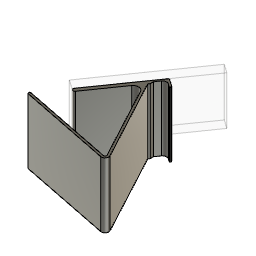
Mobilstativ v1 (Autodesk Fusion 360 design; units mm, degrees)
Autodesk Fusion 360 part; units mm, degrees
sketch "Sketch1" plane through (0, 0, 0) normal (0, 0, 1) x (1, 0, 0) in component "phone"
sketch "Sketch2" plane through (0, 0, 0) normal (0, 0, 1) x (1, 0, 0) in component "phone"
  line L0 (0, 0) -> (-28.507, 0)
  line L1 (-28.507, 0) -> (-28.507, 300.0044)
  line L2 (-28.507, 300.0044) -> (0, 300.0044)
  line L3 (0, 300.0044) -> (0, 0)
  line L4 (0, 50) -> (0, 0)
  constraint horizontal L0
  constraint vertical L1
  constraint horizontal L2
  constraint coincident L0.start L3.end
extrude "Extrude1" add sketch "Sketch2" along normal blind 40 makes body 1 in component "phone"
extrude "Extrude2" add 1 faces at (-19.0047, 116.6681, 40) along direction (0, 0, 1) blind 90 on bodies 1 bodies 1 in component "phone"
sketch "Sketch1 (2)" plane through (9.6747, 10.4809, 148.0794) normal (0, 0, 1) x (-1, 0, 0) in component "stativ"
  line L0 (68.4004, 125.7769) -> (-103.6751, -119.9723)
  line L1 (-103.6751, -119.9723) -> (-80.3235, -136.3232)
  line L2 (-80.3235, -136.3232) -> (91.7519, 109.4259)
  line L3 (91.7519, 109.4259) -> (68.4004, 125.7769)
  line L4 (65.5325, 121.6811) -> (-17.6373, 2.9023)
  line L5 (-22.9286, 12.7801) -> (-139.9865, 231.3065)
  line L6 (-129.2068, 245.8335) -> (115.8461, 196.73)
  line L7 (-17.6373, 2.9023) -> (-38.6827, -27.1535)
  line L8 (-41.4681, -27.6447) -> (-61.6426, -13.5184)
  line L9 (-25.8289, -0.0792) -> (-34.7484, -12.8175)
  line L10 (-50.0684, -15.5189) -> (-57.9556, -9.9962)
  arc A0 (-129.2068, 245.8335) -> (-139.9865, 231.3065) centre (-131.1715, 236.0284) ccw
  line L11 (-30.5905, 39.7902) -> (-134.6975, 234.1396)
  arc A1 (-130.3856, 239.9504) -> (-134.6975, 234.1396) centre (-131.1715, 236.0284) ccw
  line L12 (-130.3856, 239.9504) -> (114.6673, 190.847)
  line L13 (64.3046, 128.6448) -> (64.3046, 128.6448)
  line L14 (117.0212, 192.415) -> (117.4142, 194.376)
  arc A2 (114.6673, 190.847) -> (117.0212, 192.415) centre (115.0602, 192.808) ccw
  arc A3 (117.4142, 194.376) -> (115.8461, 196.73) centre (115.4532, 194.769) ccw
  arc A4 (64.3046, 128.6448) -> (57.341, 127.4169) centre (61.4367, 124.549) ccw
  arc A5 (65.5325, 121.6811) -> (64.3046, 128.6448) centre (61.4367, 124.549) ccw
  line L15 (-25.8289, 8.6381) -> (-25.8289, -0.0792)
  line L16 (-61.8882, -12.1256) -> (-60.7411, -10.4873)
  line L17 (57.341, 127.4169) -> (-5.0807, 38.2694)
  line L18 (-22.9286, 12.7801) -> (-25.8289, 8.6381)
  arc A6 (-50.0684, -15.5189) -> (-34.7484, -12.8175) centre (-43.759, -6.5082) ccw
  arc A7 (-41.4681, -27.6447) -> (-38.6827, -27.1535) centre (-40.321, -26.0064) ccw
  arc A8 (-57.9556, -9.9962) -> (-60.7411, -10.4873) centre (-59.1027, -11.6345) ccw
  arc A9 (-61.8882, -12.1256) -> (-61.6426, -13.5184) centre (-61.0691, -12.6992) ccw
  arc A10 (-30.5905, 39.7902) -> (-5.0807, 38.2694) centre (-17.368, 46.8731) ccw
  dimension "d9" = 10
  dimension "d10" = 2
  dimension "d11" = 5
  dimension "d12" = 11
  dimension "d13" = 2
  dimension "d14" = 2
  dimension "d15" = 1
  dimension "d16" = 15
  constraint midpoint L0 L4.end
  constraint perpendicular L7 L8
  constraint tangent L5 A0
  constraint tangent L6 A0
  constraint perpendicular L6 L14
  constraint concentric A0 A1
  constraint tangent L11 A1
  constraint tangent A1 L12
  constraint tangent L12 A2
  constraint tangent L14 A2
  constraint tangent L6 A3
  constraint tangent L14 A3
  constraint equal A2 A3
  constraint tangent A4 L17
  constraint tangent L4 A5
  constraint equal A4 A5
  constraint vertical L15
  constraint perpendicular L8 L16
  constraint coincident L5.start L17
  constraint collinear L17 L18
  constraint tangent L9 A6
  constraint tangent L10 A6
  constraint tangent L7 A7
  constraint tangent L8 A7
  constraint tangent L10 A8
  constraint tangent L16 A8
  constraint tangent L8 A9
  constraint tangent L16 A9
  constraint tangent L11 A10
  constraint tangent L17 A10
  measures "d9" radius of A0
  measures "d10" radius of A2
  measures "d11" radius of A4
  measures "d12" radius of A6
  measures "d13" radius of A7
  measures "d14" radius of A8
  measures "d15" radius of A9
  measures "d16" radius of A10
extrude "Extrude1'" add sketch "Sketch1 (2)" against normal blind 125 separate body contours L0 L4 L5 L6 L7 L8 L9 L10 A0 L11 A1 L12 L14 A2 A3 A4 A5 L15 L16 L17 L18 A6 A7 A8 A9 A10 makes body 2 in component "stativ"
extrude "Extrude2'" add 1 faces at (-4.5968, -43.8034, 23.0794) along direction (0, 0, -1) blind 50 on bodies 2 bodies 2 in component "stativ"
component "phone" placed x (0.819152, -0.573576, 0) y (0.573576, 0.819152, 0) z (0, 0, 1) at (-58.7257, -115.296, 18.0794)
component "stativ" placed x (1, 0, 0) y (0, 1, 0) z (0, 0, 1) at (0, 0, 0)
